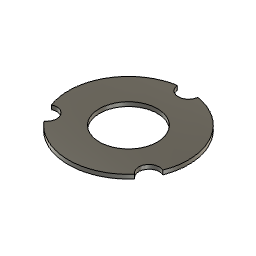
lamp reductor v1 (Autodesk Fusion 360 design; units mm, degrees)
Autodesk Fusion 360 part; units mm, degrees
sketch "Sketch1" plane through (0, 0, 0) normal (0, 0, 1) x (1, 0, 0)
  circle A0 centre (0, 0) radius 29
  circle A1 centre (0, 0) radius 14
  circle A2 centre (0.0642, 28.9999) radius 5
  circle A3 centre (24.8748, -14.9079) radius 5
  circle A4 centre (-25.0726, -14.5727) radius 5
  dimension "d1" = 58
  dimension "d2" = 28
  dimension "d3" = 10
  dimension "d4" = 10
  dimension "d5" = 10
  constraint coincident A0.centre A1.centre
  constraint concentric A0 A1
  constraint coincident A0 A2.centre
  constraint coincident A0 A3.centre
  constraint coincident A0 A4.centre
  measures "d1" diameter of A0
  measures "d2" diameter of A1
  measures "d3" diameter of A2
  measures "d4" diameter of A3
  measures "d5" diameter of A4
extrude "Extrude1" add sketch "Sketch1" along normal blind 2 contours A0 A2 A3 A4
